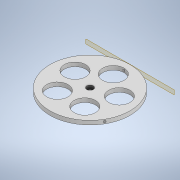
# Autodesk Inventor part: Ronde_Engine
Saved by Autodesk Inventor 2020 (Build 240168000, 168)
## iProperties
Created: 2022-04-19
Part Number: Ronde_Engine
Material: Generisch
Document SubType Name: Modeling
Designer: sp
Density: 1 g/cm^3
Appearance: Vorgabe
Author: sp
Autodesk Inventor part; units mm, degrees
ref_plane "YZ Plane" through (0, 0, 0) normal (1, 0, 0) x (0, 1, 0)
ref_plane "XZ Plane" through (0, 0, 0) normal (0, 1, 0) x (-1, 0, 0)
sketch "Skizze1" plane through (0, 0, 0) normal (0, 1, 0) x (-1, 0, 0)
  circle A0 centre (0, 0) radius 30
  dimension "d0" = 60
  constraints: 1 centre point, 1 coincident
  measures "d0" diameter of A0
extrude "Extrusion1" add sketch "Skizze1" along normal mid plane 3
sketch "Skizze2" plane through (0, 1.5, 0) normal (0, 1, 0) x (1, 0, 0)
  line L0 (0, 43.5645) -> (0, -46.3445) construction
  circle A0 centre (0, 17.5) radius 8
  circle A1 centre (-16.6435, 5.4078) radius 8
  circle A2 centre (-10.2862, -14.1578) radius 8
  circle A3 centre (10.2862, -14.1578) radius 8
  circle A4 centre (16.6435, 5.4078) radius 8
  point P0 (0, 0)
  dimension "d3" = 16
  dimension "d4" = 17.5
  dimension "d7" = 360
  constraints: 5 centre point, 2 end point, 2 point on line, 1 vertical, 11 other
  measures "d3" diameter of A0
  measures "d4" distance of point (0, 0) A0.centre
extrude "Extrusion2" cut sketch "Skizze2" against normal through all
sketch "Skizze3" plane through (0, 1.5, 0) normal (0, 1, 0) x (1, 0, 0)
  point P0 (0, 0)
  point P1 (0, 0)
  constraints: 1 coincident
hole "Bohrung1" at (0, 1.5, 0) direction (0, -1, 0) diameter 4.917 end through all thread size "M6x1" class "6H" standard "ISO Metric profile"
ref_plane "Arbeitsebene1" through (0, 0, -30) normal (0, 0, 1) x (1, 0, 0)
sketch "Skizze4" plane through (0, 0, -30) normal (0, 0, 1) x (1, 0, 0)
  point P0 (0, 0)
  point P1 (0, 0)
  constraints: 1 coincident
hole "Bohrung2" at (0, 0, -30) direction (0, 0, 1) diameter 1.567 depth 6.3 tip angle 118 thread size "M2x0.4" class "6H" standard "ISO Metric profile"
pattern_circular "Runde Anordnung1" count 3 over 360 about axis through (0, -10, 0) along (0, 1, 0) of "Bohrung2"
